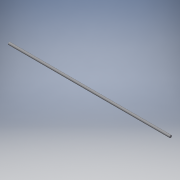
# Autodesk Inventor part: rail
Saved by Autodesk Inventor 2016 (Build 200138000, 138)
## iProperties
Created: 2017-08-15
Part Number: rail
Material: Generic
Document SubType Name: Modeling
Designer: m207653
Density: 1 g/cm^3
Appearance: Default
Author: m207653
Autodesk Inventor part; units mm, degrees
ref_plane "YZ Plane" through (0, 0, 0) normal (1, 0, 0) x (0, 1, 0)
ref_plane "XZ Plane" through (0, 0, 0) normal (0, 1, 0) x (-1, 0, 0)
ref_plane "XY Plane" through (0, 0, 0) normal (0, 0, 1) x (1, 0, 0)
sketch "Sketch1" plane through (0, 0, 0) normal (1, 0, 0) x (0, 1, 0)
  circle A0 centre (0, 0) radius 10
  dimension "d0" = 20
  constraints: 1 centre point, 1 coincident
  measures "d0" diameter of A0
extrude "Extrusion1" add sketch "Sketch1" against normal blind 1300
sketch "Sketch2" plane through (0, 0, 0) normal (1, 0, 0) x (0, 0, -1)
  circle A0 centre (0, 0) radius 10 projected
  circle A1 centre (0, 0) radius 7.5
  dimension "d5" = 15
  constraints: 1 centre point, 1 coincident
  measures "d5" diameter of A1
extrude "Extrusion2" cut sketch "Sketch2" against normal blind 1300 contours A1
sketch "Sketch4" plane through (0, 0, 0) normal (1, 0, 0) x (0, 0, -1)
  circle A0 centre (0, 0) radius 10 projected
  line L0 (0, -10) -> (10, -10)
  line L1 (10, -10) -> (10, 0)
  line L2 (10, 10) -> (-10, 10)
  line L3 (-10, 10) -> (-10, 0)
  line L4 (10, 0) -> (10, 10)
  line L5 (-10, 0) -> (-10, -10)
  line L6 (0, -10) -> (-10, -10)
  constraints: 14 end point, 5 tangent, 3 point on circle, 3 point on line, 2 horizontal, 1 parallel, 1 perpendicular
extrude "Extrusion3" add sketch "Sketch4" against normal blind 1300 contours L3 L2 A0 | A0 L6 L5 | A0 L1 L0 | L2 L4 A0
sketch "Sketch5" plane through (0, 0, 0) normal (1, 0, 0) x (0, 0, -1)
  circle A0 centre (0, 0) radius 7.5 projected
  line L0 (7.5, 0) -> (7.5, -7.5)
  line L1 (7.5, -7.5) -> (0, -7.5)
  line L2 (0, -7.5) -> (-7.5, -7.5)
  line L3 (-10, -10) -> (10, -10) projected
  line L4 (-7.5, 0) -> (-7.5, -7.5)
  line L5 (-7.5, 0) -> (-7.5, 7.5)
  line L6 (0, 7.5) -> (-7.5, 7.5)
  line L7 (0, 7.5) -> (7.5, 7.5)
  line L8 (7.5, 0) -> (7.5, 7.5)
  constraints: 16 end point, 7 tangent, 4 point on circle, 3 perpendicular, 2 vertical, 1 horizontal, 1 parallel
extrude "Extrusion4" cut sketch "Sketch5" against normal blind 1300 contours L0 L1 A0 | A0 L7 L8 | A0 L5 L6 | L2 L4 A0
body "Solid1"
